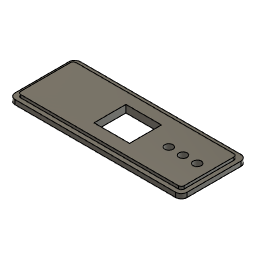
1593LBK_backplate (Autodesk Fusion 360 design; units mm, degrees)
Autodesk Fusion 360 part; units mm, degrees
sketch "Skizze1" plane through (0, 0, 0) normal (0, 1, 0) x (1, 0, 0)
  arc A0 (0, 2) -> (2, 0) centre (2, 2) ccw
  arc A1 (2, 23) -> (0, 21) centre (2, 21) ccw
  line L0 (58.5, 23) -> (2, 23)
  line L1 (60.5, 2) -> (60.5, 21)
  arc A2 (58.5, 0) -> (60.5, 2) centre (58.5, 2) ccw
  line L2 (2, 0) -> (58.5, 0)
  line L3 (0, 21) -> (0, 2)
  arc A3 (60.5, 21) -> (58.5, 23) centre (58.5, 21) ccw
  point P0 (60.5, 0)
  point P1 (0, 23)
  dimension "d1" = 60.5
  dimension "d2" = 23
  dimension "d3" = 2
  dimension "d4" = 2
  dimension "d5" = 2
  dimension "d6" = 2
  constraint horizontal L2
  constraint vertical L1
  constraint horizontal L0
  constraint vertical L3
  constraint tangent L1 A3
  constraint tangent L0 A3
  constraint coincident P0 L2
  constraint coincident P0 L1
  constraint tangent A2 L2
  constraint tangent L1 A2
  constraint coincident origin L2
  constraint coincident origin L3
  constraint tangent A0 L2
  constraint tangent A0 L3
  constraint coincident P1 L0
  constraint coincident P1 L3
  constraint tangent A1 L0
  constraint tangent A1 L3
  measures "d1" distance of origin P0
  measures "d2" distance of origin P1
  measures "d3" radius of A3
  measures "d4" radius of A2
  measures "d5" radius of A0
  measures "d6" radius of A1
sketch "Skizze2" plane through (0, 0, 0) normal (0, 1, 0) x (1, 0, 0)
  line L0 (2.5, 1.5) -> (58, 1.5)
  line L1 (59, 2.5) -> (59, 20)
  line L2 (58, 21) -> (2.5, 21)
  line L3 (1.5, 20) -> (1.5, 2.5)
  line L4 (2, 0) -> (58.5, 0)
  line L5 (0, 21) -> (0, 2)
  arc A0 (2.5, 21) -> (1.5, 20) centre (2.5, 20) ccw
  arc A1 (1.5, 2.5) -> (2.5, 1.5) centre (2.5, 2.5) ccw
  arc A2 (59, 20) -> (58, 21) centre (58, 20) ccw
  arc A3 (58, 1.5) -> (59, 2.5) centre (58, 2.5) ccw
  point P0 (1.5, 1.5)
  point P1 (59, 1.5)
  point P2 (1.5, 21)
  dimension "d7" = 57.5
  dimension "d8" = 19.5
  dimension "d9" = 1.5
  dimension "d10" = 1.5
  dimension "d11" = 1
  constraint horizontal L0
  constraint vertical L1
  constraint horizontal L2
  constraint vertical L3
  constraint coincident P2 L2
  constraint coincident P2 L3
  constraint tangent L2 A0
  constraint tangent L3 A0
  constraint coincident P0 L0
  constraint coincident P0 L3
  constraint tangent L0 A1
  constraint tangent L3 A1
  constraint equal A0 A1
  constraint tangent L1 A2
  constraint tangent L2 A2
  constraint equal A0 A2
  constraint coincident P1 L0
  constraint coincident P1 L1
  constraint tangent L0 A3
  constraint tangent L1 A3
  constraint equal A0 A3
  measures "d7" distance of P0 P1
  measures "d8" distance of P0 P2
  measures "d9" distance of L0 L4
  measures "d10" distance of L3 L5
  measures "d11" radius of A0
sketch "Skizze3" plane through (0, 0, 0) normal (0, 1, 0) x (1, 0, 0)
  line L0 (24, 17) -> (24, 5.8)
  line L1 (36.5, 17) -> (24, 17)
  line L2 (36.5, 5.8) -> (36.5, 17)
  line L3 (24, 5.8) -> (36.5, 5.8)
  line L4 (0, 21) -> (0, 2)
  line L5 (2, 0) -> (58.5, 0)
  dimension "d12" = 12.5
  dimension "d13" = 11.2
  dimension "d14" = 24
  dimension "d15" = 5.8
  constraint horizontal L3
  constraint vertical L2
  constraint horizontal L1
  constraint vertical L0
  measures "d12" distance of L2.start L0.end
  measures "d13" distance of L0.end L0.start
  measures "d14" distance of L0 L4
  measures "d15" distance of L3 L5
sketch "Skizze4" plane through (0, 0, 0) normal (0, 1, 0) x (1, 0, 0)
  circle A0 centre (44.5, 11.6) radius 1.425
  circle A1 centre (49.5, 11.6) radius 1.425
  circle A2 centre (54.5, 11.6) radius 1.425
  line L0 (2.5, 1.5) -> (58, 1.5)
  line L1 (24, 17) -> (24, 5.8)
  line L2 (36.5, 5.8) -> (36.5, 17)
  line L3 (2, 0) -> (58.5, 0)
  dimension "d16" = 2.85
  dimension "d17" = 2.85
  dimension "d18" = 2.85
  dimension "d19" = 5
  dimension "d20" = 5
  dimension "d25" = 8
  dimension "d26" = 11.6
  measures "d16" diameter of A0
  measures "d17" diameter of A1
  measures "d18" diameter of A2
  measures "d19" distance of A0.centre A1.centre
  measures "d20" distance of A1.centre A2.centre
  measures "d25" distance of A0.centre L2
  measures "d26" distance of A1.centre L3
extrude "Extrusion1" add sketch "Skizze1" along normal blind 1.6
extrude "Extrusion2" add sketch "Skizze2" along normal blind 2.6
extrude "Extrusion3" cut sketch "Skizze4" sketch "Skizze3" along normal blind 2.6 of sketch 2
equation "h1 = 3 mm"
equation "h1_hoehe = 6.5 mm"
